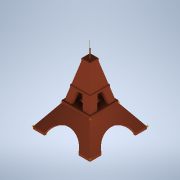
# Autodesk Inventor part: torre
Saved by Autodesk Inventor 2021 (Build 250183000, 183)
## iProperties
Created: 2021-06-14
Part Number: torre
Material: Genérico
Document SubType Name: Modeling
Designer: yosaf
Density: 1 g/cm^3
Appearance: Valor por defecto
Author: yosaf
Autodesk Inventor part; units mm, degrees
sketch "Boceto1" plane through (0, 0, 0) normal (0, 1, 0) x (-1, 0, 0)
  line L0 (12.5, 12.5) -> (-12.5, 12.5)
  line L1 (-12.5, 12.5) -> (-12.5, -12.5)
  line L2 (-12.5, -12.5) -> (12.5, -12.5)
  line L3 (12.5, -12.5) -> (12.5, 12.5)
  line L4 (3.75, -3.75) -> (-3.75, -3.75)
  line L5 (-3.75, -3.75) -> (-3.75, 3.75)
  line L6 (-3.75, 3.75) -> (3.75, 3.75)
  line L7 (3.75, 3.75) -> (3.75, -3.75)
  point P0 (0, 0)
  dimension "d0" = 25
  dimension "d1" = 25
  dimension "d2" = 12.5
  dimension "d3" = 12.5
  dimension "d9" = 7.5
  dimension "d10" = 7.5
  dimension "d11" = 3.75
  dimension "d12" = 3.75
  constraints: 16 end point, 4 parallel, 2 horizontal, 2 perpendicular
  measures "d0" distance of L2.end L1.end
  measures "d1" distance of L1.end L0.end
  measures "d2" horizontal distance of point (0, 0) L2.end
  measures "d3" horizontal distance of L2.end point (0, 0)
  measures "d9" distance of L5.end L6.end
  measures "d10" distance of L4.end L5.end
  measures "d11" horizontal distance of point (0, 0) L4.start
  measures "d12" horizontal distance of L4.start point (0, 0)
extrude "Extrusión1" add sketch "Boceto1" along normal blind 2 contours L3 L2 L1 L0 | L4 L5 L6 L7
ref_plane "Plano de trabajo1" through (0, -20, 0) normal (0, -1, 0) x (1, 0, 0)
ref_plane "Plano de trabajo2" through (0, 32, 0) normal (0, 1, 0) x (1, 0, 0)
ref_plane "Plano de trabajo3" through (0, 12, 0) normal (0, 1, 0) x (1, 0, 0)
sketch "Boceto2" plane through (0, 2, 0) normal (0, 1, 0) x (1, 0, 0)
  line L0 (-5, 5) -> (5, 5)
  line L1 (5, 5) -> (5, -5)
  line L2 (5, -5) -> (-5, -5)
  line L3 (-5, -5) -> (-5, 5)
  point P0 (0, 0)
  dimension "d13" = 5
  dimension "d14" = 10
  dimension "d15" = 5
  dimension "d16" = 10
  constraints: 8 end point, 2 parallel, 1 horizontal, 1 perpendicular
  measures "d13" horizontal distance of L0.start point (0, 0)
  measures "d14" distance of L0.end L0.start
  measures "d15" horizontal distance of L0.start point (0, 0)
  measures "d16" distance of L0.start L2.end
extrude "Extrusión2" cut sketch "Boceto2" against normal blind 2
sketch "Boceto3" plane through (0, -20, 0) normal (0, -1, 0) x (1, 0, 0)
  line L0 (-25, 25) -> (25, 25)
  line L1 (25, 25) -> (25, -25)
  line L2 (25, -25) -> (-25, -25)
  line L3 (-25, -25) -> (-25, 25)
  line L4 (-23, 23) -> (23, 23)
  line L5 (23, 23) -> (23, -23)
  line L6 (23, -23) -> (-23, -23)
  line L7 (-23, -23) -> (-23, 23)
  line L8 (-15, 25) -> (-15, 23)
  line L9 (-25, 15) -> (-23, 15)
  line L10 (15, 25) -> (15, 23)
  line L11 (25, 15) -> (23, 15)
  line L12 (-15, -25) -> (-15, -23)
  line L13 (-25, -15) -> (-23, -15)
  line L14 (25, -15) -> (23, -15)
  line L15 (15, -25) -> (15, -23)
  point P0 (0, 0)
  dimension "d19" = 50
  dimension "d20" = 50
  dimension "d21" = 25
  dimension "d22" = 25
  dimension "d23" = 46
  dimension "d24" = 46
  dimension "d25" = 23
  dimension "d26" = 23
  constraints: 32 end point, 18 point on line, 8 perpendicular, 4 parallel, 2 horizontal
  measures "d19" distance of L1.end L2.end
  measures "d20" distance of L0.end L1.end
  measures "d21" horizontal distance of L0.start point (0, 0)
  measures "d22" horizontal distance of L0.start point (0, 0)
  measures "d23" distance of L5.end L6.end
  measures "d24" distance of L4.end L5.end
  measures "d25" horizontal distance of point (0, 0) L4.start
  measures "d26" horizontal distance of point (0, 0) L4.start
extrude "Extrusión3" add sketch "Boceto3" against normal blind 2 contours L0 L8 L4 L7 L9 L3 | L0 L1 L11 L5 L4 L10 | L13 L7 L6 L12 L2 L3 | L1 L2 L15 L6 L5 L14
ref_plane "Plano de trabajo4" through (12.5, 0, -12.5) normal (0, -0.57, 0.8216) x (-1, 0, 0)
sketch "Boceto4" plane through (12.5, 0, -12.5) normal (0, -0.57, 0.8216) x (-1, 0, 0)
  line L0 (-12.5, 21.9146) -> (-2.5, 21.9146) projected
  line L1 (37.5, 21.9146) -> (37.5, 16.2146) projected
  line L2 (25, 0) -> (25, -14.2499) projected
  arc A0 (-2.5, 21.9146) -> (27.5, 21.9146) centre (12.5, 26.7031) ccw
  line L3 (-2.5, 21.9146) -> (-12.5, 21.9146)
  line L4 (-12.5, 17.8579) -> (-12.5, 16.2146) projected
  line L5 (0, 0) -> (0, -1.6433) projected
  line L6 (27.5, 21.9146) -> (37.5, 21.9146)
  line L7 (35.5, -0.8853) -> (37.5, -0.8853) projected
  line L8 (37.5, 21.9146) -> (23.6374, -2.4057)
  line L9 (-12.5, 21.9146) -> (1.3799, -2.4057)
  line L10 (1.3799, -2.4057) -> (23.6374, -2.4057)
  point P0 (12.5, -7.125)
  dimension "d30" = 15.7458
  constraints: 10 end point, 2 perpendicular, 2 point on circle, 1 centre point, 1 parallel, 1 point on line
  measures "d30" radius of A0
extrude "Extrusión4" add sketch "Boceto4" along normal blind 2
pattern_circular "Patrón circular1" count 4 over 360 about axis through (0, -10, 0) along (0, 1, 0) of "Extrusión4"
sketch "Boceto5" plane through (0, 12, 0) normal (0, 1, 0) x (1, 0, 0)
  line L0 (5, 5) -> (-5, 5) projected
  line L1 (5, -5) -> (5, 5) projected
  line L2 (-5, 5) -> (5, 5)
  line L3 (5, 5) -> (5, -5)
  line L4 (5, -5) -> (-5, -5)
  line L5 (-5, -5) -> (-5, 5)
  line L6 (-8.75, 8.75) -> (8.75, 8.75)
  line L7 (8.75, 8.75) -> (8.75, -8.75)
  line L8 (8.75, -8.75) -> (-8.75, -8.75)
  line L9 (-8.75, -8.75) -> (-8.75, 8.75)
  point P0 (0, 0)
  dimension "d36" = 17.5
  dimension "d37" = 17.5
  dimension "d38" = 8.75
  dimension "d39" = 8.75
  constraints: 16 end point, 4 parallel, 2 horizontal, 2 perpendicular
  measures "d36" distance of L7.end L8.end
  measures "d37" distance of L6.end L7.end
  measures "d38" horizontal distance of point (0, 0) L8.end
  measures "d39" horizontal distance of point (0, 0) L6.end
extrude "Extrusión5" add sketch "Boceto5" along normal blind 2
ref_plane "Plano de trabajo5" through (-8.75, 12, 8.75) normal (0, 0.2419, 0.9703) x (1, 0, 0)
sketch "Boceto6" plane through (-8.75, 12, 8.75) normal (0, 0.2419, 0.9703) x (1, 0, 0)
  line L0 (-3.75, -6.5092) -> (-3.75, -12.5508) projected
  line L1 (-3.75, -10.3116) -> (21.2497, -10.3116)
  line L2 (-3.75, -12.5508) -> (-2.4955, -10.3116)
  line L3 (21.2497, -10.3116) -> (19.9947, -10.3116)
  line L4 (-2.4955, -10.3116) -> (0.467, 1.9406)
  line L5 (0, 1.9406) -> (17.5, 1.9406) projected
  line L6 (19.9947, -10.3116) -> (17.0283, 1.9406)
  line L7 (0.4668, 1.9398) -> (17.0284, 1.9398)
  line L8 (0.4668, 1.9398) -> (17.0284, 1.9398) construction
  line L9 (-2.4955, -10.3116) -> (3.7545, -10.3116)
  line L10 (0, 0) -> (17.5, 0) projected
  line L11 (8.75, 0) -> (6.75, 0)
  line L12 (6.75, 0) -> (3.7545, -10.3116)
  line L13 (8.75, 0) -> (10.75, 0)
  line L14 (19.9947, -10.3116) -> (13.7447, -10.3116)
  line L15 (13.7447, -10.3116) -> (10.75, 0)
  point P0 (8.75, -9.5267)
  dimension "d43" = 1.2545
  dimension "d44" = 1.255
  dimension "d45" = 0
  dimension "d46" = 6.25
  dimension "d47" = 2
  dimension "d48" = 2
  dimension "d49" = 6.25
  constraints: 26 end point, 11 point on line, 2 horizontal, 1 collinear, 1 midpoint
  measures "d43" distance of L2.end L1.start
  measures "d44" distance of L1.end L3.end
  measures "d45" distance between parallel lines of L7 L8
  measures "d46" distance of L2.end L9.end
  measures "d47" distance of L11.start L11.end
  measures "d48" distance of L11.start L13.end
  measures "d49" distance of L3.end L14.end
extrude "Extrusión6" add sketch "Boceto6" against normal blind 2 contours L4 L5 L6 L10 L12 L1 | L15 L10 L6 L1
pattern_circular "Patrón circular2" count 4 over 360 about axis through (0, -10, 0) along (0, 1, 0) of "Extrusión6"
sketch "Boceto7" plane through (0, 32, 0) normal (0, 1, 0) x (1, 0, 0)
  line L0 (-3.75, -3.75) -> (3.75, -3.75)
  line L1 (3.75, -3.75) -> (3.75, 3.75)
  line L2 (3.75, 3.75) -> (-3.75, 3.75)
  line L3 (-3.75, 3.75) -> (-3.75, -3.75)
  point P0 (0, 0)
  dimension "d55" = 7.5
  dimension "d56" = 7.5
  constraints: 8 end point, 2 parallel, 1 horizontal, 1 perpendicular
  measures "d55" distance of L2.end L1.end
  measures "d56" distance of L1.end L0.end
extrude "Extrusión7" add sketch "Boceto7" along normal blind 2
ref_plane "Plano de trabajo6" through (3.75, 32, 3.75) normal (0.9703, 0.2419, 0) x (0, 0, -1)
sketch "Boceto8" plane through (3.75, 32, 3.75) normal (0.9703, 0.2419, 0) x (0, 0, -1)
  line L0 (-5, -14.4413) -> (-5, -18.6749) projected
  line L1 (-5, -18.5577) -> (12.5036, -18.5577)
  line L2 (0, 0) -> (7.5, 0) projected
  line L3 (0, 0) -> (7.5, 0)
  line L4 (14.9785, -30.9217) -> (12.4622, -20.6155) projected
  line L5 (12.4622, -20.6155) -> (11.9437, -18.5577)
  line L6 (11.9437, -18.5577) -> (12.5036, -18.5577)
  line L7 (12.5036, -18.5577) -> (12.0036, -18.5577)
  line L8 (-5, -18.5577) -> (-4.5, -18.5577)
  line L9 (-4.5, -18.5577) -> (0.4628, 1.8839)
  line L10 (12.0036, -18.5577) -> (7.0641, 1.7766)
  line L11 (7.1342, 1.4879) -> (0.3667, 1.4879)
  point P0 (3.75, -30.1423)
  point P1 (12.0036, -18.5577)
  dimension "d60" = 0.5
  dimension "d61" = 0.5
  constraints: 18 end point, 8 point on line, 2 collinear, 1 horizontal, 1 perpendicular
  measures "d60" distance of L1.end L7.end
  measures "d61" distance of L1.start L8.end
extrude "Extrusión8" add sketch "Boceto8" against normal blind 2
pattern_circular "Patrón circular3" count 4 over 360 about axis through (0, -10, 0) along (0, 1, 0) of "Extrusión8"
ref_plane "Plano de trabajo7" through (1.6888, 32, -1.6888) normal (0, 1, 0) x (1, 0, 0)
sketch "Boceto9" plane through (0, 34, 0) normal (0, 1, 0) x (1, 0, 0)
  circle A0 centre (0, 0) radius 0.5
  dimension "d67" = 1
  constraints: 1 centre point, 1 coincident
  measures "d67" diameter of A0
extrude "Extrusión9" add sketch "Boceto9" along normal blind 7.5
